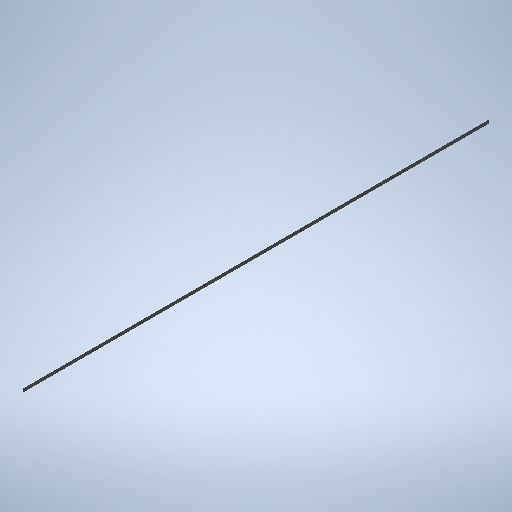
# Autodesk Inventor part: JUNTA DE FELPA 3000 mm
Saved by Autodesk Inventor 2025 (Build 290162000, 162)
## iProperties
Created: 2026-02-24
Part Number: JUNTA DE FELPA 3000 mm
Material: Caucho
Document SubType Name: Modeling
Designer: Frank
Density: 0.93 g/cm^3
Appearance: Suave - Gris claro
Author: Frank
Autodesk Inventor part; units mm, degrees
ref_plane "YZ Plane" through (0, 0, 0) normal (1, 0, 0) x (0, 1, 0)
ref_plane "XZ Plane" through (0, 0, 0) normal (0, 1, 0) x (-1, 0, 0)
ref_plane "XY Plane" through (0, 0, 0) normal (0, 0, 1) x (1, 0, 0)
sketch "Boceto1" plane through (0, 0, 0) normal (0, 0, 1) x (1, 0, 0)
  line L0 (-18.4596, -13.534) -> (-18.4596, -15.934)
  line L1 (-18.4596, -15.934) -> (-19.8596, -15.934)
  line L2 (-19.8596, -15.934) -> (-19.8596, -13.934)
  line L3 (-19.8596, -13.934) -> (-21.3596, -13.934)
  line L4 (-21.3596, -13.934) -> (-21.3596, -21.934)
  line L5 (-21.3596, -21.934) -> (-19.8596, -21.934)
  line L6 (-19.8596, -21.934) -> (-19.8596, -19.934)
  line L7 (-19.8596, -19.934) -> (-18.4596, -19.934)
  line L8 (-18.4596, -19.934) -> (-18.4596, -22.334)
  line L9 (-18.4596, -13.534) -> (-16.4596, -13.534)
  line L10 (-16.4596, -13.534) -> (-16.4596, -22.334)
  line L11 (-16.4596, -22.334) -> (-18.4596, -22.334)
  point P0 (-26.2596, -17.734)
  point P1 (-21.3596, -17.934)
  dimension "d28" = 1.4
  dimension "d30" = 1.4
  dimension "d34" = 8
  dimension "d35" = 2
  dimension "d36" = 4
  dimension "d37" = 1.5
  dimension "d64" = 8.8
  dimension "d65" = 2
  constraints: 24 end point, 8 perpendicular, 1 horizontal, 1 midpoint, 1 point on line, 1 vertical
  measures "d28" distance between parallel lines of L0 L2
  measures "d30" distance between parallel lines of L8 L6
  measures "d34" distance between parallel lines of L5 L3
  measures "d35" distance from line of L1 point (-21.36, -17.934)
  measures "d36" distance between parallel lines of L7 L1
  measures "d37" distance between parallel lines of L4 L2
  measures "d64" distance of L9.end L10.end
  measures "d65" distance of L0.start L9.end
extrude "Extrusión1" add sketch "Boceto1" along normal blind 3000
